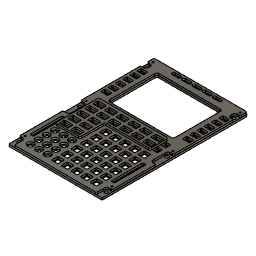
MCDU (3D layered extrusion based on SVG) (Autodesk Fusion 360 design; units mm, degrees)
Autodesk Fusion 360 part; units mm, degrees
(part 1 of 3)
sketch "Bottom" plane through (0, 0, 0) normal (0, 0, 1) x (1, 0, 0)
  ellipse E0 centre (25.7081, -64.7405) end of major axis (27.0103, -64.7405) minor radius 1.2936 (25.7081, -66.0341) -> (24.4058, -64.7405) cw
  line L0 (25.7081, -66.0341) -> (36.7769, -66.0341)
  ellipse E1 centre (36.7769, -64.7405) end of major axis (38.0792, -64.7405) minor radius 1.2936 (38.0792, -64.7405) -> (36.7769, -66.0341) cw
  line L1 (38.0792, -64.7405) -> (38.0792, -58.6604)
  ellipse E2 centre (36.7769, -58.6604) end of major axis (38.0792, -58.6604) minor radius 1.2936 (36.7769, -57.3667) -> (38.0792, -58.6604) cw
  line L2 (36.7769, -57.3667) -> (25.7081, -57.3667)
  ellipse E3 centre (25.7081, -58.6604) end of major axis (27.0103, -58.6604) minor radius 1.2936 (24.4058, -58.6604) -> (25.7081, -57.3667) cw
  line L3 (24.4058, -58.6604) -> (24.4058, -64.7405)
  ellipse E4 centre (25.7081, -75.9348) end of major axis (27.0103, -75.9348) minor radius 1.2936 (25.7081, -77.2285) -> (24.4058, -75.9348) cw
  line L4 (25.7081, -77.2285) -> (36.7769, -77.2285)
  ellipse E5 centre (36.7769, -75.9348) end of major axis (38.0792, -75.9348) minor radius 1.2936 (38.0792, -75.9348) -> (36.7769, -77.2285) cw
  line L5 (38.0792, -75.9348) -> (38.0792, -69.8548)
  ellipse E6 centre (36.7769, -69.8548) end of major axis (38.0792, -69.8548) minor radius 1.2936 (36.7769, -68.5611) -> (38.0792, -69.8548) cw
  line L6 (36.7769, -68.5611) -> (25.7081, -68.5611)
  ellipse E7 centre (25.7081, -69.8548) end of major axis (27.0103, -69.8548) minor radius 1.2936 (24.4058, -69.8548) -> (25.7081, -68.5611) cw
  line L7 (24.4058, -69.8548) -> (24.4058, -75.9348)
  ellipse E8 centre (25.7081, -87.174) end of major axis (27.0103, -87.174) minor radius 1.2936 (25.7081, -88.4676) -> (24.4058, -87.174) cw
  line L8 (25.7081, -88.4676) -> (36.7769, -88.4676)
  ellipse E9 centre (36.7769, -87.174) end of major axis (38.0792, -87.174) minor radius 1.2936 (38.0792, -87.174) -> (36.7769, -88.4676) cw
  line L9 (38.0792, -87.174) -> (38.0792, -81.0939)
  ellipse E10 centre (36.7769, -81.0939) end of major axis (38.0792, -81.0939) minor radius 1.2936 (36.7769, -79.8003) -> (38.0792, -81.0939) cw
  line L10 (36.7769, -79.8003) -> (25.7081, -79.8003)
  ellipse E11 centre (25.7081, -81.0939) end of major axis (27.0103, -81.0939) minor radius 1.2936 (24.4058, -81.0939) -> (25.7081, -79.8003) cw
  line L11 (24.4058, -81.0939) -> (24.4058, -87.174)
  ellipse E12 centre (25.7081, -98.4373) end of major axis (27.0103, -98.4373) minor radius 1.2936 (25.7081, -99.7309) -> (24.4058, -98.4373) cw
  line L12 (25.7081, -99.7309) -> (36.7769, -99.7309)
  ellipse E13 centre (36.7769, -98.4373) end of major axis (38.0792, -98.4373) minor radius 1.2936 (38.0792, -98.4373) -> (36.7769, -99.7309) cw
  line L13 (38.0792, -98.4373) -> (38.0792, -92.3572)
  ellipse E14 centre (36.7769, -92.3572) end of major axis (38.0792, -92.3572) minor radius 1.2936 (36.7769, -91.0636) -> (38.0792, -92.3572) cw
  line L14 (36.7769, -91.0636) -> (25.7081, -91.0636)
  ellipse E15 centre (25.7081, -92.3572) end of major axis (27.0103, -92.3572) minor radius 1.2936 (24.4058, -92.3572) -> (25.7081, -91.0636) cw
  line L15 (24.4058, -92.3572) -> (24.4058, -98.4373)
  ellipse E16 centre (25.7081, -109.6497) end of major axis (27.0103, -109.6497) minor radius 1.2936 (25.7081, -110.9433) -> (24.4058, -109.6497) cw
  line L16 (25.7081, -110.9433) -> (36.7769, -110.9433)
  ellipse E17 centre (36.7769, -109.6497) end of major axis (38.0792, -109.6497) minor radius 1.2936 (38.0792, -109.6497) -> (36.7769, -110.9433) cw
  line L17 (38.0792, -109.6497) -> (38.0792, -103.5696)
  ellipse E18 centre (36.7769, -103.5696) end of major axis (38.0792, -103.5696) minor radius 1.2936 (36.7769, -102.276) -> (38.0792, -103.5696) cw
  line L18 (36.7769, -102.276) -> (25.7081, -102.276)
  ellipse E19 centre (25.7081, -103.5696) end of major axis (27.0103, -103.5696) minor radius 1.2936 (24.4058, -103.5696) -> (25.7081, -102.276) cw
  line L19 (24.4058, -103.5696) -> (24.4058, -109.6497)
  ellipse E20 centre (25.7081, -120.8865) end of major axis (27.0103, -120.8865) minor radius 1.2936 (25.7081, -122.1801) -> (24.4058, -120.8865) cw
  line L20 (25.7081, -122.1801) -> (36.7769, -122.1801)
  ellipse E21 centre (36.7769, -120.8865) end of major axis (38.0792, -120.8865) minor radius 1.2936 (38.0792, -120.8865) -> (36.7769, -122.1801) cw
  line L21 (38.0792, -120.8865) -> (38.0792, -114.8064)
  ellipse E22 centre (36.7769, -114.8064) end of major axis (38.0792, -114.8064) minor radius 1.2936 (36.7769, -113.5127) -> (38.0792, -114.8064) cw
  line L22 (36.7769, -113.5127) -> (25.7081, -113.5127)
  ellipse E23 centre (25.7081, -114.8064) end of major axis (27.0103, -114.8064) minor radius 1.2936 (24.4058, -114.8064) -> (25.7081, -113.5127) cw
  line L23 (24.4058, -114.8064) -> (24.4058, -120.8865)
  ellipse E24 centre (153.6745, -120.9659) end of major axis (154.9767, -120.9659) minor radius 1.2936 (153.6745, -122.2596) -> (152.3723, -120.9659) cw
  line L24 (153.6745, -122.2596) -> (164.7434, -122.2596)
  ellipse E25 centre (164.7434, -120.9659) end of major axis (166.0456, -120.9659) minor radius 1.2936 (166.0456, -120.9659) -> (164.7434, -122.2596) cw
  line L25 (166.0456, -120.9659) -> (166.0456, -114.8858)
  ellipse E26 centre (164.7434, -114.8858) end of major axis (166.0456, -114.8858) minor radius 1.2936 (164.7434, -113.5922) -> (166.0456, -114.8858) cw
  line L26 (164.7434, -113.5922) -> (153.6745, -113.5922)
  ellipse E27 centre (153.6745, -114.8858) end of major axis (154.9767, -114.8858) minor radius 1.2936 (152.3723, -114.8858) -> (153.6745, -113.5922) cw
  line L27 (152.3723, -114.8858) -> (152.3723, -120.9659)
  ellipse E28 centre (153.6745, -98.4902) end of major axis (154.9767, -98.4902) minor radius 1.2936 (153.6745, -99.7839) -> (152.3723, -98.4902) cw
  line L28 (153.6745, -99.7839) -> (164.7434, -99.7839)
  ellipse E29 centre (164.7434, -98.4902) end of major axis (166.0456, -98.4902) minor radius 1.2936 (166.0456, -98.4902) -> (164.7434, -99.7839) cw
  line L29 (166.0456, -98.4902) -> (166.0456, -92.4102)
  ellipse E30 centre (164.7434, -92.4102) end of major axis (166.0456, -92.4102) minor radius 1.2936 (164.7434, -91.1165) -> (166.0456, -92.4102) cw
  line L30 (164.7434, -91.1165) -> (153.6745, -91.1165)
  ellipse E31 centre (153.6745, -92.4102) end of major axis (154.9767, -92.4102) minor radius 1.2936 (152.3723, -92.4102) -> (153.6745, -91.1165) cw
  line L31 (152.3723, -92.4102) -> (152.3723, -98.4902)
  ellipse E32 centre (153.6745, -87.28) end of major axis (154.9767, -87.28) minor radius 1.2936 (153.6745, -88.5736) -> (152.3723, -87.28) cw
  line L32 (153.6745, -88.5736) -> (164.7434, -88.5736)
  ellipse E33 centre (164.7434, -87.28) end of major axis (166.0456, -87.28) minor radius 1.2936 (166.0456, -87.28) -> (164.7434, -88.5736) cw
  line L33 (166.0456, -87.28) -> (166.0456, -81.1999)
  ellipse E34 centre (164.7434, -81.1999) end of major axis (166.0456, -81.1999) minor radius 1.2936 (164.7434, -79.9062) -> (166.0456, -81.1999) cw
  line L34 (164.7434, -79.9062) -> (153.6745, -79.9062)
  ellipse E35 centre (153.6745, -81.1999) end of major axis (154.9767, -81.1999) minor radius 1.2936 (152.3723, -81.1999) -> (153.6745, -79.9062) cw
  line L35 (152.3723, -81.1999) -> (152.3723, -87.28)
  ellipse E36 centre (153.6745, -76.0143) end of major axis (154.9767, -76.0143) minor radius 1.2936 (153.6745, -77.308) -> (152.3723, -76.0143) cw
  line L36 (153.6745, -77.308) -> (164.7434, -77.308)
  ellipse E37 centre (164.7434, -76.0143) end of major axis (166.0456, -76.0143) minor radius 1.2936 (166.0456, -76.0143) -> (164.7434, -77.308) cw
  line L37 (166.0456, -76.0143) -> (166.0456, -69.9342)
  ellipse E38 centre (164.7434, -69.9342) end of major axis (166.0456, -69.9342) minor radius 1.2936 (164.7434, -68.6406) -> (166.0456, -69.9342) cw
  line L38 (164.7434, -68.6406) -> (153.6745, -68.6406)
  ellipse E39 centre (153.6745, -69.9342) end of major axis (154.9767, -69.9342) minor radius 1.2936 (152.3723, -69.9342) -> (153.6745, -68.6406) cw
  line L39 (152.3723, -69.9342) -> (152.3723, -76.0143)
  ellipse E40 centre (153.6748, -64.7405) end of major axis (154.977, -64.7405) minor radius 1.2936 (153.6748, -66.0341) -> (152.3726, -64.7405) cw
  line L40 (153.6748, -66.0341) -> (164.7437, -66.0341)
  ellipse E41 centre (164.7437, -64.7405) end of major axis (166.0459, -64.7405) minor radius 1.2936 (166.0459, -64.7405) -> (164.7437, -66.0341) cw
  line L41 (166.0459, -64.7405) -> (166.0459, -58.6604)
  ellipse E42 centre (164.7437, -58.6604) end of major axis (166.0459, -58.6604) minor radius 1.2936 (164.7437, -57.3667) -> (166.0459, -58.6604) cw
  line L42 (164.7437, -57.3667) -> (153.6748, -57.3667)
  ellipse E43 centre (153.6748, -58.6604) end of major axis (154.977, -58.6604) minor radius 1.2936 (152.3726, -58.6604) -> (153.6748, -57.3667) cw
  line L43 (152.3726, -58.6604) -> (152.3726, -64.7405)
  ellipse E44 centre (39.5473, -146.6503) end of major axis (40.6602, -146.6503) minor radius 1.1983 (39.5473, -147.8487) -> (38.4344, -146.6503) cw
  line L44 (39.5473, -147.8487) -> (52.0339, -147.8487)
  ellipse E45 centre (52.0339, -146.6503) end of major axis (53.1468, -146.6503) minor radius 1.1983 (53.1468, -146.6503) -> (52.0339, -147.8487) cw
  line L45 (53.1468, -146.6503) -> (53.1468, -139.3406)
  ellipse E46 centre (52.0339, -139.3406) end of major axis (53.1468, -139.3406) minor radius 1.1983 (52.0339, -138.1423) -> (53.1468, -139.3406) cw
  line L46 (52.0339, -138.1423) -> (39.5473, -138.1423)
  ellipse E47 centre (39.5473, -139.3406) end of major axis (40.6602, -139.3406) minor radius 1.1983 (38.4344, -139.3406) -> (39.5473, -138.1423) cw
  line L47 (38.4344, -139.3406) -> (38.4344, -146.6503)
  ellipse E48 centre (39.5473, -159.4672) end of major axis (40.6602, -159.4672) minor radius 1.1983 (39.5473, -160.6656) -> (38.4344, -159.4672) cw
  line L48 (39.5473, -160.6656) -> (52.0339, -160.6656)
  ellipse E49 centre (52.0339, -159.4672) end of major axis (53.1468, -159.4672) minor radius 1.1983 (53.1468, -159.4672) -> (52.0339, -160.6656) cw
  line L49 (53.1468, -159.4672) -> (53.1468, -152.1575)
  ellipse E50 centre (52.0339, -152.1575) end of major axis (53.1468, -152.1575) minor radius 1.1983 (52.0339, -150.9592) -> (53.1468, -152.1575) cw
  line L50 (52.0339, -150.9592) -> (39.5473, -150.9592)
  ellipse E51 centre (39.5473, -152.1575) end of major axis (40.6602, -152.1575) minor radius 1.1983 (38.4344, -152.1575) -> (39.5473, -150.9592) cw
  line L51 (38.4344, -152.1575) -> (38.4344, -159.4672)
  ellipse E52 centre (39.5473, -172.8669) end of major axis (40.6602, -172.8669) minor radius 1.1983 (39.5473, -174.0652) -> (38.4344, -172.8669) cw
  line L52 (39.5473, -174.0652) -> (52.0339, -174.0652)
  ellipse E53 centre (52.0339, -172.8669) end of major axis (53.1468, -172.8669) minor radius 1.1983 (53.1468, -172.8669) -> (52.0339, -174.0652) cw
  line L53 (53.1468, -172.8669) -> (53.1468, -165.5572)
  ellipse E54 centre (52.0339, -165.5572) end of major axis (53.1468, -165.5572) minor radius 1.1983 (52.0339, -164.3588) -> (53.1468, -165.5572) cw
  line L54 (52.0339, -164.3588) -> (39.5473, -164.3588)
  ellipse E55 centre (39.5473, -165.5572) end of major axis (40.6602, -165.5572) minor radius 1.1983 (38.4344, -165.5572) -> (39.5473, -164.3588) cw
  line L55 (38.4344, -165.5572) -> (38.4344, -172.8669)
  ellipse E56 centre (39.5473, -185.9547) end of major axis (40.6602, -185.9547) minor radius 1.1983 (39.5473, -187.1531) -> (38.4344, -185.9547) cw
  line L56 (39.5473, -187.1531) -> (52.0339, -187.1531)
  ellipse E57 centre (52.0339, -185.9547) end of major axis (53.1468, -185.9547) minor radius 1.1983 (53.1468, -185.9547) -> (52.0339, -187.1531) cw
  line L57 (53.1468, -185.9547) -> (53.1468, -178.645)
  ellipse E58 centre (52.0339, -178.645) end of major axis (53.1468, -178.645) minor radius 1.1983 (52.0339, -177.4467) -> (53.1468, -178.645) cw
  line L58 (52.0339, -177.4467) -> (39.5473, -177.4466)
  ellipse E59 centre (39.5473, -178.645) end of major axis (40.6602, -178.645) minor radius 1.1983 (38.4344, -178.645) -> (39.5473, -177.4466) cw
  line L59 (38.4344, -178.645) -> (38.4344, -185.9547)
  ellipse E60 centre (39.5473, -198.9895) end of major axis (40.6602, -198.9895) minor radius 1.1983 (39.5473, -200.1878) -> (38.4344, -198.9895) cw
  line L60 (39.5473, -200.1878) -> (52.0339, -200.1878)
  ellipse E61 centre (52.0339, -198.9895) end of major axis (53.1468, -198.9895) minor radius 1.1983 (53.1468, -198.9895) -> (52.0339, -200.1878) cw
  line L61 (53.1468, -198.9895) -> (53.1468, -191.6797)
  ellipse E62 centre (52.0339, -191.6797) end of major axis (53.1468, -191.6797) minor radius 1.1983 (52.0339, -190.4814) -> (53.1468, -191.6797) cw
  line L62 (52.0339, -190.4814) -> (39.5473, -190.4814)
  ellipse E63 centre (39.5473, -191.6797) end of major axis (40.6602, -191.6797) minor radius 1.1983 (38.4344, -191.6797) -> (39.5473, -190.4814) cw
  line L63 (38.4344, -191.6797) -> (38.4344, -198.9895)
  ellipse E64 centre (57.4439, -198.9895) end of major axis (58.5568, -198.9895) minor radius 1.1983 (57.4439, -200.1878) -> (56.331, -198.9895) cw
  line L64 (57.4439, -200.1878) -> (69.9305, -200.1878)
  ellipse E65 centre (69.9305, -198.9895) end of major axis (71.0434, -198.9895) minor radius 1.1983 (71.0434, -198.9895) -> (69.9305, -200.1878) cw
  line L65 (71.0434, -198.9895) -> (71.0434, -191.6797)
  ellipse E66 centre (69.9305, -191.6797) end of major axis (71.0434, -191.6797) minor radius 1.1983 (69.9305, -190.4814) -> (71.0434, -191.6797) cw
  line L66 (69.9305, -190.4814) -> (57.4439, -190.4814)
  ellipse E67 centre (57.4439, -191.6797) end of major axis (58.5568, -191.6797) minor radius 1.1983 (56.331, -191.6797) -> (57.4439, -190.4814) cw
  line L67 (56.331, -191.6797) -> (56.331, -198.9895)
  ellipse E68 centre (57.4439, -185.9547) end of major axis (58.5568, -185.9547) minor radius 1.1983 (57.4439, -187.1531) -> (56.331, -185.9547) cw
  line L68 (57.4439, -187.1531) -> (69.9305, -187.1531)
  ellipse E69 centre (69.9305, -185.9547) end of major axis (71.0434, -185.9547) minor radius 1.1983 (71.0434, -185.9547) -> (69.9305, -187.1531) cw
  line L69 (71.0434, -185.9547) -> (71.0434, -178.645)
  ellipse E70 centre (69.9305, -178.645) end of major axis (71.0434, -178.645) minor radius 1.1983 (69.9305, -177.4467) -> (71.0434, -178.645) cw
  line L70 (69.9305, -177.4467) -> (57.4439, -177.4466)
  ellipse E71 centre (57.4439, -178.645) end of major axis (58.5568, -178.645) minor radius 1.1983 (56.331, -178.645) -> (57.4439, -177.4466) cw
  line L71 (56.331, -178.645) -> (56.331, -185.9547)
  ellipse E72 centre (57.4439, -172.8669) end of major axis (58.5568, -172.8669) minor radius 1.1983 (57.4439, -174.0652) -> (56.331, -172.8669) cw
  line L72 (57.4439, -174.0652) -> (69.9305, -174.0652)
  ellipse E73 centre (69.9305, -172.8669) end of major axis (71.0434, -172.8669) minor radius 1.1983 (71.0434, -172.8669) -> (69.9305, -174.0652) cw
  line L73 (71.0434, -172.8669) -> (71.0434, -165.5572)
  ellipse E74 centre (69.9305, -165.5572) end of major axis (71.0434, -165.5572) minor radius 1.1983 (69.9305, -164.3588) -> (71.0434, -165.5572) cw
  line L74 (69.9305, -164.3588) -> (57.4439, -164.3588)
  ellipse E75 centre (57.4439, -165.5572) end of major axis (58.5568, -165.5572) minor radius 1.1983 (56.331, -165.5572) -> (57.4439, -164.3588) cw
  line L75 (56.331, -165.5572) -> (56.331, -172.8669)
  ellipse E76 centre (57.4439, -159.4672) end of major axis (58.5568, -159.4672) minor radius 1.1983 (57.4439, -160.6656) -> (56.331, -159.4672) cw
  line L76 (57.4439, -160.6656) -> (69.9305, -160.6656)
  ellipse E77 centre (69.9305, -159.4672) end of major axis (71.0434, -159.4672) minor radius 1.1983 (71.0434, -159.4672) -> (69.9305, -160.6656) cw
  line L77 (71.0434, -159.4672) -> (71.0434, -152.1575)
  ellipse E78 centre (69.9305, -152.1575) end of major axis (71.0434, -152.1575) minor radius 1.1983 (69.9305, -150.9592) -> (71.0434, -152.1575) cw
  line L78 (69.9305, -150.9592) -> (57.4439, -150.9592)
  ellipse E79 centre (57.4439, -152.1575) end of major axis (58.5568, -152.1575) minor radius 1.1983 (56.331, -152.1575) -> (57.4439, -150.9592) cw
  line L79 (56.331, -152.1575) -> (56.331, -159.4672)
  ellipse E80 centre (57.4439, -146.6503) end of major axis (58.5568, -146.6503) minor radius 1.1983 (57.4439, -147.8487) -> (56.331, -146.6503) cw
  line L80 (57.4439, -147.8487) -> (69.9305, -147.8487)
  ellipse E81 centre (69.9305, -146.6503) end of major axis (71.0434, -146.6503) minor radius 1.1983 (71.0434, -146.6503) -> (69.9305, -147.8487) cw
  line L81 (71.0434, -146.6503) -> (71.0434, -139.3406)
  ellipse E82 centre (69.9305, -139.3406) end of major axis (71.0434, -139.3406) minor radius 1.1983 (69.9305, -138.1423) -> (71.0434, -139.3406) cw
  line L82 (69.9305, -138.1423) -> (57.4439, -138.1423)
  ellipse E83 centre (57.4439, -139.3406) end of major axis (58.5568, -139.3406) minor radius 1.1983 (56.331, -139.3406) -> (57.4439, -138.1423) cw
  line L83 (56.331, -139.3406) -> (56.331, -146.6503)
  ellipse E84 centre (75.6043, -146.6503) end of major axis (76.7172, -146.6503) minor radius 1.1983 (75.6044, -147.8487) -> (74.4915, -146.6503) cw
  line L84 (75.6044, -147.8487) -> (88.091, -147.8487)
  ellipse E85 centre (88.0909, -146.6503) end of major axis (89.2038, -146.6503) minor radius 1.1983 (89.2038, -146.6503) -> (88.091, -147.8487) cw
  line L85 (89.2038, -146.6503) -> (89.2038, -139.3406)
  ellipse E86 centre (88.0909, -139.3406) end of major axis (89.2038, -139.3406) minor radius 1.1983 (88.091, -138.1423) -> (89.2038, -139.3406) cw
  line L86 (88.091, -138.1423) -> (75.6044, -138.1423)
  ellipse E87 centre (75.6043, -139.3406) end of major axis (76.7172, -139.3406) minor radius 1.1983 (74.4915, -139.3406) -> (75.6044, -138.1423) cw
  line L87 (74.4915, -139.3406) -> (74.4915, -146.6503)
  ellipse E88 centre (75.6043, -159.4672) end of major axis (76.7172, -159.4672) minor radius 1.1983 (75.6044, -160.6656) -> (74.4915, -159.4672) cw
  line L88 (75.6044, -160.6656) -> (88.091, -160.6656)
  ellipse E89 centre (88.0909, -159.4672) end of major axis (89.2038, -159.4672) minor radius 1.1983 (89.2038, -159.4672) -> (88.091, -160.6656) cw
  line L89 (89.2038, -159.4672) -> (89.2038, -152.1575)
  ellipse E90 centre (88.0909, -152.1575) end of major axis (89.2038, -152.1575) minor radius 1.1983 (88.091, -150.9592) -> (89.2038, -152.1575) cw
  line L90 (88.091, -150.9592) -> (75.6044, -150.9592)
  ellipse E91 centre (75.6043, -152.1575) end of major axis (76.7172, -152.1575) minor radius 1.1983 (74.4915, -152.1575) -> (75.6044, -150.9592) cw
  line L91 (74.4915, -152.1575) -> (74.4915, -159.4672)
  ellipse E92 centre (93.7913, -146.6503) end of major axis (94.9042, -146.6503) minor radius 1.1983 (93.7913, -147.8487) -> (92.6784, -146.6503) cw
  line L92 (93.7913, -147.8487) -> (106.2779, -147.8487)
  ellipse E93 centre (106.2779, -146.6503) end of major axis (107.3908, -146.6503) minor radius 1.1983 (107.3908, -146.6503) -> (106.2779, -147.8487) cw
  line L93 (107.3908, -146.6503) -> (107.3908, -139.3406)
  ellipse E94 centre (106.2779, -139.3406) end of major axis (107.3908, -139.3406) minor radius 1.1983 (106.2779, -138.1423) -> (107.3908, -139.3406) cw
  line L94 (106.2779, -138.1423) -> (93.7913, -138.1423)
  ellipse E95 centre (93.7913, -139.3406) end of major axis (94.9042, -139.3406) minor radius 1.1983 (92.6784, -139.3406) -> (93.7913, -138.1423) cw
  line L95 (92.6784, -139.3406) -> (92.6784, -146.6503)
  ellipse E96 centre (93.7913, -159.4672) end of major axis (94.9042, -159.4672) minor radius 1.1983 (93.7913, -160.6656) -> (92.6784, -159.4672) cw
  line L96 (93.7913, -160.6656) -> (106.2779, -160.6656)
  ellipse E97 centre (106.2779, -159.4672) end of major axis (107.3908, -159.4672) minor radius 1.1983 (107.3908, -159.4672) -> (106.2779, -160.6656) cw
  line L97 (107.3908, -159.4672) -> (107.3908, -152.1575)
  ellipse E98 centre (106.2779, -152.1575) end of major axis (107.3908, -152.1575) minor radius 1.1983 (106.2779, -150.9592) -> (107.3908, -152.1575) cw
  line L98 (106.2779, -150.9592) -> (93.7913, -150.9592)
  ellipse E99 centre (93.7913, -152.1575) end of major axis (94.9042, -152.1575) minor radius 1.1983 (92.6784, -152.1575) -> (93.7913, -150.9592) cw
  line L99 (92.6784, -152.1575) -> (92.6784, -159.4672)
  ellipse E100 centre (111.7928, -146.6503) end of major axis (112.9057, -146.6503) minor radius 1.1983 (111.7928, -147.8487) -> (110.6799, -146.6503) cw
  line L100 (111.7928, -147.8487) -> (124.2794, -147.8487)
  ellipse E101 centre (124.2794, -146.6503) end of major axis (125.3923, -146.6503) minor radius 1.1983 (125.3923, -146.6503) -> (124.2794, -147.8487) cw
  line L101 (125.3923, -146.6503) -> (125.3923, -139.3406)
  ellipse E102 centre (124.2794, -139.3406) end of major axis (125.3923, -139.3406) minor radius 1.1983 (124.2794, -138.1423) -> (125.3923, -139.3406) cw
  line L102 (124.2794, -138.1423) -> (111.7928, -138.1423)
  ellipse E103 centre (111.7928, -139.3406) end of major axis (112.9057, -139.3406) minor radius 1.1983 (110.6799, -139.3406) -> (111.7928, -138.1423) cw
  line L103 (110.6799, -139.3406) -> (110.6799, -146.6503)
  ellipse E104 centre (111.7928, -159.4672) end of major axis (112.9057, -159.4672) minor radius 1.1983 (111.7928, -160.6656) -> (110.6799, -159.4672) cw
  line L104 (111.7928, -160.6656) -> (124.2794, -160.6656)
  ellipse E105 centre (124.2794, -159.4672) end of major axis (125.3923, -159.4672) minor radius 1.1983 (125.3923, -159.4672) -> (124.2794, -160.6656) cw
  line L105 (125.3923, -159.4672) -> (125.3923, -152.1575)
  ellipse E106 centre (124.2794, -152.1575) end of major axis (125.3923, -152.1575) minor radius 1.1983 (124.2794, -150.9592) -> (125.3923, -152.1575) cw
  line L106 (124.2794, -150.9592) -> (111.7928, -150.9592)
  ellipse E107 centre (111.7928, -152.1575) end of major axis (112.9057, -152.1575) minor radius 1.1983 (110.6799, -152.1575) -> (111.7928, -150.9592) cw
  line L107 (110.6799, -152.1575) -> (110.6799, -159.4672)
  ellipse E108 centre (129.7572, -146.6503) end of major axis (130.8701, -146.6503) minor radius 1.1983 (129.7572, -147.8487) -> (128.6444, -146.6503) cw
  line L108 (129.7572, -147.8487) -> (142.2439, -147.8487)
  ellipse E109 centre (142.2439, -146.6503) end of major axis (143.3567, -146.6503) minor radius 1.1983 (143.3567, -146.6503) -> (142.2439, -147.8487) cw
  line L109 (143.3567, -146.6503) -> (143.3567, -139.3406)
  ellipse E110 centre (142.2439, -139.3406) end of major axis (143.3567, -139.3406) minor radius 1.1983 (142.2439, -138.1423) -> (143.3567, -139.3406) cw
  line L110 (142.2439, -138.1423) -> (129.7573, -138.1423)
  ellipse E111 centre (129.7573, -139.3406) end of major axis (130.8701, -139.3406) minor radius 1.1983 (128.6444, -139.3406) -> (129.7573, -138.1423) cw
  line L111 (128.6444, -139.3406) -> (128.6444, -146.6503)
  ellipse E112 centre (129.7572, -159.4672) end of major axis (130.8701, -159.4672) minor radius 1.1983 (129.7572, -160.6656) -> (128.6444, -159.4672) cw
  line L112 (129.7572, -160.6656) -> (142.2439, -160.6656)
  ellipse E113 centre (142.2439, -159.4672) end of major axis (143.3567, -159.4672) minor radius 1.1983 (143.3567, -159.4672) -> (142.2439, -160.6656) cw
  line L113 (143.3567, -159.4672) -> (143.3567, -152.1575)
  ellipse E114 centre (142.2439, -152.1575) end of major axis (143.3567, -152.1575) minor radius 1.1983 (142.2439, -150.9592) -> (143.3567, -152.1575) cw
  line L114 (142.2439, -150.9592) -> (129.7573, -150.9592)
  ellipse E115 centre (129.7573, -152.1575) end of major axis (130.8701, -152.1575) minor radius 1.1983 (128.6444, -152.1575) -> (129.7573, -150.9592) cw
  line L115 (128.6444, -152.1575) -> (128.6444, -159.4672)
  arc A0 (125.3436, -178.7576) -> (124.0756, -177.4896) centre (125.3436, -177.4896) cw
  line L116 (125.3436, -178.7576) -> (135.4877, -178.7576)
  arc A1 (136.7557, -177.4896) -> (135.4877, -178.7576) centre (135.4877, -177.4896) cw
  line L117 (136.7557, -177.4896) -> (136.7557, -167.3456)
  arc A2 (135.4877, -166.0776) -> (136.7557, -167.3456) centre (135.4877, -167.3456) cw
  line L118 (135.4877, -166.0776) -> (125.3436, -166.0776)
  arc A3 (124.0756, -167.3456) -> (125.3436, -166.0776) centre (125.3436, -167.3456) cw
  line L119 (124.0756, -167.3456) -> (124.0756, -177.4896)
  arc A4 (140.3318, -178.7166) -> (139.0637, -177.4486) centre (140.3317, -177.4486) cw
  line L120 (140.3318, -178.7166) -> (150.4758, -178.7166)
  arc A5 (151.7438, -177.4486) -> (150.4758, -178.7166) centre (150.4758, -177.4486) cw
  line L121 (151.7438, -177.4486) -> (151.7438, -167.3045)
  arc A6 (150.4758, -166.0365) -> (151.7438, -167.3045) centre (150.4758, -167.3045) cw
  line L122 (150.4758, -166.0365) -> (140.3318, -166.0365)
  arc A7 (139.0638, -167.3045) -> (140.3318, -166.0365) centre (140.3318, -167.3045) cw
  line L123 (139.0638, -167.3045) -> (139.0637, -177.4486)
  arc A8 (80.0241, -178.7576) -> (78.7561, -177.4896) centre (80.0241, -177.4896) cw
  line L124 (80.0241, -178.7576) -> (90.1681, -178.7576)
  arc A9 (91.4361, -177.4896) -> (90.1681, -178.7576) centre (90.1681, -177.4896) cw
  line L125 (91.4361, -177.4896) -> (91.4361, -167.3456)
  arc A10 (90.1681, -166.0776) -> (91.4361, -167.3456) centre (90.1681, -167.3456) cw
  line L126 (90.1681, -166.0776) -> (80.0241, -166.0776)
  arc A11 (78.7561, -167.3456) -> (80.0241, -166.0776) centre (80.0241, -167.3456) cw
  line L127 (78.7561, -167.3456) -> (78.7561, -177.4896)
  arc A12 (95.0489, -178.7576) -> (93.7809, -177.4896) centre (95.0489, -177.4896) cw
  line L128 (95.0489, -178.7576) -> (105.193, -178.7576)
  arc A13 (106.461, -177.4896) -> (105.193, -178.7576) centre (105.193, -177.4896) cw
  line L129 (106.461, -177.4896) -> (106.461, -167.3456)
  arc A14 (105.193, -166.0776) -> (106.461, -167.3456) centre (105.193, -167.3456) cw
  line L130 (105.193, -166.0776) -> (95.0489, -166.0776)
  arc A15 (93.7809, -167.3456) -> (95.0489, -166.0776) centre (95.0489, -167.3456) cw
  line L131 (93.7809, -167.3456) -> (93.7809, -177.4896)
  arc A16 (110.2136, -178.7576) -> (108.9456, -177.4896) centre (110.2136, -177.4896) cw
  line L132 (110.2136, -178.7576) -> (120.3577, -178.7576)
  arc A17 (121.6257, -177.4896) -> (120.3577, -178.7576) centre (120.3577, -177.4896) cw
  line L133 (121.6257, -177.4896) -> (121.6257, -167.3456)
  arc A18 (120.3577, -166.0776) -> (121.6257, -167.3456) centre (120.3577, -167.3456) cw
  line L134 (120.3577, -166.0776) -> (110.2136, -166.0776)
  arc A19 (108.9456, -167.3456) -> (110.2136, -166.0776) centre (110.2136, -167.3456) cw
  line L135 (108.9456, -167.3456) -> (108.9456, -177.4896)
  arc A20 (140.3318, -193.6928) -> (139.0637, -192.4248) centre (140.3317, -192.4248) cw
  line L136 (140.3318, -193.6928) -> (150.4758, -193.6928)
  arc A21 (151.7438, -192.4248) -> (150.4758, -193.6928) centre (150.4758, -192.4248) cw
  line L137 (151.7438, -192.4248) -> (151.7438, -182.2807)
  arc A22 (150.4758, -181.0127) -> (151.7438, -182.2807) centre (150.4758, -182.2807) cw
  line L138 (150.4758, -181.0127) -> (140.3318, -181.0127)
  arc A23 (139.0638, -182.2807) -> (140.3318, -181.0127) centre (140.3318, -182.2807) cw
  line L139 (139.0638, -182.2807) -> (139.0637, -192.4248)
  arc A24 (125.3436, -193.7338) -> (124.0756, -192.4658) centre (125.3436, -192.4658) cw
  line L140 (125.3436, -193.7338) -> (135.4877, -193.7338)
  arc A25 (136.7557, -192.4658) -> (135.4877, -193.7338) centre (135.4877, -192.4658) cw
  line L141 (136.7557, -192.4658) -> (136.7557, -182.3218)
  arc A26 (135.4877, -181.0538) -> (136.7557, -182.3218) centre (135.4877, -182.3218) cw
  line L142 (135.4877, -181.0538) -> (125.3436, -181.0538)
  arc A27 (124.0756, -182.3218) -> (125.3436, -181.0538) centre (125.3436, -182.3218) cw
  line L143 (124.0756, -182.3218) -> (124.0756, -192.4658)
  arc A28 (110.2136, -193.7338) -> (108.9456, -192.4658) centre (110.2136, -192.4658) cw
  line L144 (110.2136, -193.7338) -> (120.3577, -193.7338)
  arc A29 (121.6257, -192.4658) -> (120.3577, -193.7338) centre (120.3577, -192.4658) cw
  line L145 (121.6257, -192.4658) -> (121.6257, -182.3218)
  arc A30 (120.3577, -181.0538) -> (121.6257, -182.3218) centre (120.3577, -182.3218) cw
  line L146 (120.3577, -181.0538) -> (110.2136, -181.0538)
  arc A31 (108.9456, -182.3218) -> (110.2136, -181.0538) centre (110.2136, -182.3218) cw
  line L147 (108.9456, -182.3218) -> (108.9456, -192.4658)
  arc A32 (95.0489, -193.7338) -> (93.7809, -192.4658) centre (95.0489, -192.4658) cw
  line L148 (95.0489, -193.7338) -> (105.193, -193.7338)
  arc A33 (106.461, -192.4658) -> (105.193, -193.7338) centre (105.193, -192.4658) cw
  line L149 (106.461, -192.4658) -> (106.461, -182.3218)
  arc A34 (105.193, -181.0538) -> (106.461, -182.3218) centre (105.193, -182.3218) cw
  line L150 (105.193, -181.0538) -> (95.0489, -181.0538)
  arc A35 (93.7809, -182.3218) -> (95.0489, -181.0538) centre (95.0489, -182.3218) cw
  line L151 (93.7809, -182.3218) -> (93.7809, -192.4658)
  arc A36 (80.0241, -193.7338) -> (78.7561, -192.4658) centre (80.0241, -192.4658) cw
  line L152 (80.0241, -193.7338) -> (90.1681, -193.7338)
  arc A37 (91.4361, -192.4658) -> (90.1681, -193.7338) centre (90.1681, -192.4658) cw
  line L153 (91.4361, -192.4658) -> (91.4361, -182.3218)
  arc A38 (90.1681, -181.0538) -> (91.4361, -182.3218) centre (90.1681, -182.3218) cw
  line L154 (90.1681, -181.0538) -> (80.0241, -181.0538)
  arc A39 (78.7561, -182.3218) -> (80.0241, -181.0538) centre (80.0241, -182.3218) cw
  line L155 (78.7561, -182.3218) -> (78.7561, -192.4658)
  arc A40 (140.3318, -208.7485) -> (139.0638, -207.4805) centre (140.3318, -207.4805) cw
  line L156 (140.3318, -208.7485) -> (150.4758, -208.7485)
  arc A41 (151.7438, -207.4805) -> (150.4758, -208.7485) centre (150.4758, -207.4805) cw
  line L157 (151.7438, -207.4805) -> (151.7438, -197.3365)
  arc A42 (150.4758, -196.0685) -> (151.7438, -197.3365) centre (150.4758, -197.3365) cw
  line L158 (150.4758, -196.0685) -> (140.3318, -196.0685)
  arc A43 (139.0638, -197.3365) -> (140.3318, -196.0685) centre (140.3318, -197.3365) cw
  line L159 (139.0638, -197.3365) -> (139.0638, -207.4805)
  arc A44 (125.3436, -208.7896) -> (124.0756, -207.5215) centre (125.3436, -207.5216) cw
  line L160 (125.3436, -208.7896) -> (135.4877, -208.7896)
  arc A45 (136.7557, -207.5215) -> (135.4877, -208.7896) centre (135.4877, -207.5216) cw
  line L161 (136.7557, -207.5215) -> (136.7557, -197.3775)
  arc A46 (135.4877, -196.1095) -> (136.7557, -197.3775) centre (135.4877, -197.3775) cw
  line L162 (135.4877, -196.1095) -> (125.3436, -196.1095)
  arc A47 (124.0756, -197.3775) -> (125.3436, -196.1095) centre (125.3436, -197.3775) cw
  line L163 (124.0756, -197.3775) -> (124.0756, -207.5215)
  arc A48 (110.2136, -208.7896) -> (108.9456, -207.5215) centre (110.2136, -207.5216) cw
  line L164 (110.2136, -208.7896) -> (120.3577, -208.7896)
  arc A49 (121.6257, -207.5215) -> (120.3577, -208.7896) centre (120.3577, -207.5216) cw
  line L165 (121.6257, -207.5215) -> (121.6257, -197.3775)
  arc A50 (120.3577, -196.1095) -> (121.6257, -197.3775) centre (120.3577, -197.3775) cw
  line L166 (120.3577, -196.1095) -> (110.2136, -196.1095)
  arc A51 (108.9456, -197.3775) -> (110.2136, -196.1095) centre (110.2136, -197.3775) cw
  line L167 (108.9456, -197.3775) -> (108.9456, -207.5215)
  arc A52 (95.0489, -208.7896) -> (93.7809, -207.5215) centre (95.0489, -207.5216) cw
  line L168 (95.0489, -208.7896) -> (105.193, -208.7896)
  arc A53 (106.461, -207.5215) -> (105.193, -208.7896) centre (105.193, -207.5216) cw
  line L169 (106.461, -207.5215) -> (106.461, -197.3775)
  arc A54 (105.193, -196.1095) -> (106.461, -197.3775) centre (105.193, -197.3775) cw
  line L170 (105.193, -196.1095) -> (95.0489, -196.1095)
  arc A55 (93.7809, -197.3775) -> (95.0489, -196.1095) centre (95.0489, -197.3775) cw
  line L171 (93.7809, -197.3775) -> (93.7809, -207.5215)
  arc A56 (80.0241, -208.7896) -> (78.7561, -207.5215) centre (80.0241, -207.5216) cw
  line L172 (80.0241, -208.7896) -> (90.1681, -208.7896)
  arc A57 (91.4361, -207.5215) -> (90.1681, -208.7896) centre (90.1681, -207.5216) cw
  line L173 (91.4361, -207.5215) -> (91.4361, -197.3775)
  arc A58 (90.1681, -196.1095) -> (91.4361, -197.3775) centre (90.1681, -197.3775) cw
  line L174 (90.1681, -196.1095) -> (80.0241, -196.1095)
  arc A59 (78.7561, -197.3775) -> (80.0241, -196.1095) centre (80.0241, -197.3775) cw
  line L175 (78.7561, -197.3775) -> (78.7561, -207.5215)
  arc A60 (140.3318, -223.7776) -> (139.0638, -222.5096) centre (140.3318, -222.5096) cw
  line L176 (140.3318, -223.7776) -> (150.4758, -223.7776)
  arc A61 (151.7438, -222.5096) -> (150.4758, -223.7776) centre (150.4758, -222.5096) cw
  line L177 (151.7438, -222.5096) -> (151.7438, -212.3655)
  arc A62 (150.4758, -211.0975) -> (151.7438, -212.3655) centre (150.4758, -212.3655) cw
  line L178 (150.4758, -211.0975) -> (140.3318, -211.0975)
  arc A63 (139.0638, -212.3655) -> (140.3318, -211.0975) centre (140.3318, -212.3655) cw
  line L179 (139.0638, -212.3655) -> (139.0638, -222.5096)
  arc A64 (125.3436, -223.8186) -> (124.0756, -222.5506) centre (125.3436, -222.5506) cw
  line L180 (125.3436, -223.8186) -> (135.4877, -223.8186)
  arc A65 (136.7557, -222.5506) -> (135.4877, -223.8186) centre (135.4877, -222.5506) cw
  line L181 (136.7557, -222.5506) -> (136.7557, -212.4066)
  arc A66 (135.4877, -211.1386) -> (136.7557, -212.4066) centre (135.4877, -212.4066) cw
  line L182 (135.4877, -211.1386) -> (125.3436, -211.1386)
  arc A67 (124.0756, -212.4066) -> (125.3436, -211.1386) centre (125.3436, -212.4066) cw
  line L183 (124.0756, -212.4066) -> (124.0756, -222.5506)
  arc A68 (110.2136, -223.8186) -> (108.9456, -222.5506) centre (110.2136, -222.5506) cw
  line L184 (110.2136, -223.8186) -> (120.3577, -223.8186)
  arc A69 (121.6257, -222.5506) -> (120.3577, -223.8186) centre (120.3577, -222.5506) cw
  line L185 (121.6257, -222.5506) -> (121.6257, -212.4066)
  arc A70 (120.3577, -211.1386) -> (121.6257, -212.4066) centre (120.3577, -212.4066) cw
  line L186 (120.3577, -211.1386) -> (110.2136, -211.1386)
  arc A71 (108.9456, -212.4066) -> (110.2136, -211.1386) centre (110.2136, -212.4066) cw
  line L187 (108.9456, -212.4066) -> (108.9456, -222.5506)
  arc A72 (95.0489, -223.8186) -> (93.7809, -222.5506) centre (95.0489, -222.5506) cw
  line L188 (95.0489, -223.8186) -> (105.193, -223.8186)
  arc A73 (106.461, -222.5506) -> (105.193, -223.8186) centre (105.193, -222.5506) cw
  line L189 (106.461, -222.5506) -> (106.461, -212.4066)
  arc A74 (105.193, -211.1386) -> (106.461, -212.4066) centre (105.193, -212.4066) cw
  line L190 (105.193, -211.1386) -> (95.0489, -211.1386)
  arc A75 (93.7809, -212.4066) -> (95.0489, -211.1386) centre (95.0489, -212.4066) cw
  line L191 (93.7809, -212.4066) -> (93.7809, -222.5506)
  arc A76 (80.0241, -223.8186) -> (78.7561, -222.5506) centre (80.0241, -222.5506) cw
  line L192 (80.0241, -223.8186) -> (90.1681, -223.8186)
  arc A77 (91.4361, -222.5506) -> (90.1681, -223.8186) centre (90.1681, -222.5506) cw
  line L193 (91.4361, -222.5506) -> (91.4361, -212.4066)
  arc A78 (90.1681, -211.1386) -> (91.4361, -212.4066) centre (90.1681, -212.4066) cw
  line L194 (90.1681, -211.1386) -> (80.0241, -211.1386)
  arc A79 (78.7561, -212.4066) -> (80.0241, -211.1386) centre (80.0241, -212.4066) cw
  line L195 (78.7561, -212.4066) -> (78.7561, -222.5506)
  arc A80 (140.3317, -238.8069) -> (139.0637, -237.5389) centre (140.3317, -237.5389) cw
  line L196 (140.3317, -238.8069) -> (150.4758, -238.8069)
  arc A81 (151.7438, -237.5389) -> (150.4758, -238.8069) centre (150.4758, -237.5389) cw
  line L197 (151.7438, -237.5389) -> (151.7438, -227.3949)
  arc A82 (150.4758, -226.1269) -> (151.7438, -227.3949) centre (150.4758, -227.3949) cw
  line L198 (150.4758, -226.1269) -> (140.3317, -226.1269)
  arc A83 (139.0637, -227.3949) -> (140.3317, -226.1269) centre (140.3317, -227.3949) cw
  line L199 (139.0637, -227.3949) -> (139.0637, -237.5389)
  arc A84 (125.3436, -238.848) -> (124.0756, -237.58) centre (125.3436, -237.58) cw
  line L200 (125.3436, -238.848) -> (135.4877, -238.848)
  arc A85 (136.7557, -237.58) -> (135.4877, -238.848) centre (135.4877, -237.58) cw
  line L201 (136.7557, -237.58) -> (136.7557, -227.4359)
  arc A86 (135.4877, -226.1679) -> (136.7557, -227.4359) centre (135.4877, -227.4359) cw
  line L202 (135.4877, -226.1679) -> (125.3436, -226.1679)
  arc A87 (124.0756, -227.436) -> (125.3436, -226.1679) centre (125.3436, -227.4359) cw
  line L203 (124.0756, -227.436) -> (124.0756, -237.58)
  arc A88 (110.2136, -238.848) -> (108.9456, -237.58) centre (110.2136, -237.58) cw
  line L204 (110.2136, -238.848) -> (120.3577, -238.848)
  arc A89 (121.6257, -237.58) -> (120.3577, -238.848) centre (120.3577, -237.58) cw
  line L205 (121.6257, -237.58) -> (121.6257, -227.4359)
  arc A90 (120.3577, -226.1679) -> (121.6257, -227.4359) centre (120.3577, -227.4359) cw
  line L206 (120.3577, -226.1679) -> (110.2136, -226.1679)
  arc A91 (108.9456, -227.436) -> (110.2136, -226.1679) centre (110.2136, -227.4359) cw
  line L207 (108.9456, -227.436) -> (108.9456, -237.58)
  arc A92 (95.0489, -238.848) -> (93.7809, -237.58) centre (95.0489, -237.58) cw
  line L208 (95.0489, -238.848) -> (105.193, -238.848)
  arc A93 (106.461, -237.58) -> (105.193, -238.848) centre (105.193, -237.58) cw
  line L209 (106.461, -237.58) -> (106.461, -227.4359)
  arc A94 (105.193, -226.1679) -> (106.461, -227.4359) centre (105.193, -227.4359) cw
  line L210 (105.193, -226.1679) -> (95.0489, -226.1679)
  arc A95 (93.7809, -227.436) -> (95.0489, -226.1679) centre (95.0489, -227.4359) cw
  line L211 (93.7809, -227.436) -> (93.7809, -237.58)
  arc A96 (80.0241, -238.848) -> (78.7561, -237.58) centre (80.0241, -237.58) cw
  line L212 (80.0241, -238.848) -> (90.1681, -238.848)
  arc A97 (91.4361, -237.58) -> (90.1681, -238.848) centre (90.1681, -237.58) cw
  line L213 (91.4361, -237.58) -> (91.4361, -227.4359)
  arc A98 (90.1681, -226.1679) -> (91.4361, -227.4359) centre (90.1681, -227.4359) cw
  line L214 (90.1681, -226.1679) -> (80.0241, -226.1679)
  arc A99 (78.7561, -227.436) -> (80.0241, -226.1679) centre (80.0241, -227.4359) cw
  line L215 (78.7561, -227.436) -> (78.7561, -237.58)
  arc A100 (140.3318, -253.889) -> (139.0638, -252.621) centre (140.3318, -252.621) cw
  line L216 (140.3318, -253.889) -> (150.4758, -253.889)
  arc A101 (151.7438, -252.6209) -> (150.4758, -253.889) centre (150.4758, -252.621) cw
  line L217 (151.7438, -252.6209) -> (151.7438, -242.4769)
  arc A102 (150.4758, -241.2089) -> (151.7438, -242.4769) centre (150.4758, -242.477) cw
  line L218 (150.4758, -241.2089) -> (140.3318, -241.2089)
  arc A103 (139.0638, -242.4769) -> (140.3318, -241.2089) centre (140.3318, -242.477) cw
  line L219 (139.0638, -242.4769) -> (139.0638, -252.621)
  arc A104 (125.3436, -253.9301) -> (124.0756, -252.662) centre (125.3436, -252.662) cw
  line L220 (125.3436, -253.9301) -> (135.4877, -253.9301)
  arc A105 (136.7557, -252.662) -> (135.4877, -253.9301) centre (135.4877, -252.662) cw
  line L221 (136.7557, -252.662) -> (136.7557, -242.518)
  arc A106 (135.4877, -241.25) -> (136.7557, -242.518) centre (135.4877, -242.518) cw
  line L222 (135.4877, -241.25) -> (125.3436, -241.25)
  arc A107 (124.0756, -242.518) -> (125.3436, -241.25) centre (125.3436, -242.518) cw
  line L223 (124.0756, -242.518) -> (124.0756, -252.662)
  arc A108 (110.2136, -253.9301) -> (108.9456, -252.662) centre (110.2136, -252.662) cw
  line L224 (110.2136, -253.9301) -> (120.3577, -253.9301)
  arc A109 (121.6257, -252.662) -> (120.3577, -253.9301) centre (120.3577, -252.662) cw
  line L225 (121.6257, -252.662) -> (121.6257, -242.518)
  arc A110 (120.3577, -241.25) -> (121.6257, -242.518) centre (120.3577, -242.518) cw
  line L226 (120.3577, -241.25) -> (110.2136, -241.25)
  arc A111 (108.9456, -242.518) -> (110.2136, -241.25) centre (110.2136, -242.518) cw
  line L227 (108.9456, -242.518) -> (108.9456, -252.662)
  arc A112 (95.0489, -253.9301) -> (93.7809, -252.662) centre (95.0489, -252.662) cw
  line L228 (95.0489, -253.9301) -> (105.193, -253.9301)
  arc A113 (106.461, -252.662) -> (105.193, -253.9301) centre (105.193, -252.662) cw
  line L229 (106.461, -252.662) -> (106.461, -242.518)
  arc A114 (105.193, -241.25) -> (106.461, -242.518) centre (105.193, -242.518) cw
  line L230 (105.193, -241.25) -> (95.0489, -241.25)
  arc A115 (93.7809, -242.518) -> (95.0489, -241.25) centre (95.0489, -242.518) cw
  line L231 (93.7809, -242.518) -> (93.7809, -252.662)
  arc A116 (80.0241, -253.9301) -> (78.756, -252.662) centre (80.0241, -252.662) cw
  line L232 (80.0241, -253.9301) -> (90.1681, -253.9301)
  arc A117 (91.4361, -252.662) -> (90.1681, -253.9301) centre (90.1681, -252.662) cw
  line L233 (91.4361, -252.662) -> (91.4361, -242.518)
  arc A118 (90.1681, -241.25) -> (91.4361, -242.518) centre (90.1681, -242.518) cw
  line L234 (90.1681, -241.25) -> (80.0241, -241.25)
  arc A119 (78.756, -242.518) -> (80.0241, -241.25) centre (80.0241, -242.518) cw
  line L235 (78.756, -242.518) -> (78.756, -252.662)
  arc A120 (160.8405, -250.3707) -> (165.8205, -250.3707) centre (163.3305, -250.3681) cw
  arc A121 (165.8205, -250.3707) -> (160.8405, -250.3707) centre (163.3305, -250.3734) cw
  ellipse E116 centre (26.873, -250.3909) end of major axis (29.3663, -250.3909) minor radius 2.492 (29.3663, -250.3909) -> (24.3798, -250.3909) cw
  ellipse E117 centre (26.873, -250.3909) end of major axis (29.3663, -250.3909) minor radius 2.492 (24.3798, -250.3909) -> (29.3663, -250.3909) cw
  ellipse E118 centre (163.3052, -155.0041) end of major axis (165.7973, -155.0041) minor radius 2.4899 (165.7973, -155.0041) -> (160.8131, -155.0041) cw
  ellipse E119 centre (163.3052, -155.0041) end of major axis (165.7973, -155.0041) minor radius 2.4899 (160.8131, -155.0041) -> (165.7973, -155.0041) cw
  arc A122 (24.3761, -154.9952) -> (29.3602, -154.9952) centre (26.8681, -154.9941) cw
  arc A123 (29.3602, -154.9952) -> (24.3761, -154.9952) centre (26.8681, -154.9963) cw
  ellipse E120 centre (163.2903, -50.1084) end of major axis (165.7824, -50.1084) minor radius 2.4899 (160.7982, -50.1106) -> (165.7824, -50.1106) cw
  ellipse E121 centre (163.2903, -50.1128) end of major axis (165.7824, -50.1128) minor radius 2.4899 (165.7824, -50.1106) -> (160.7982, -50.1106) cw
  ellipse E122 centre (26.863, -50.1096) end of major axis (29.3551, -50.1096) minor radius 2.4913 (24.371, -50.112) -> (29.3551, -50.112) cw
  ellipse E123 centre (26.863, -50.1145) end of major axis (29.3551, -50.1145) minor radius 2.4913 (29.3551, -50.112) -> (24.371, -50.112) cw
  ellipse E124 centre (153.6745, -109.7292) end of major axis (154.9767, -109.7292) minor radius 1.2936 (153.6745, -111.0228) -> (152.3723, -109.7291) cw
  line L236 (153.6745, -111.0228) -> (164.7434, -111.0228)
  ellipse E125 centre (164.7434, -109.7292) end of major axis (166.0456, -109.7292) minor radius 1.2936 (166.0456, -109.7291) -> (164.7434, -111.0228) cw
  line L237 (166.0456, -109.7291) -> (166.0456, -103.6491)
  ellipse E126 centre (164.7434, -103.6491) end of major axis (166.0456, -103.6491) minor radius 1.2936 (164.7434, -102.3554) -> (166.0456, -103.6491) cw
  line L238 (164.7434, -102.3554) -> (153.6745, -102.3554)
  ellipse E127 centre (153.6745, -103.6491) end of major axis (154.9767, -103.6491) minor radius 1.2936 (152.3723, -103.6491) -> (153.6745, -102.3554) cw
  line L239 (152.3723, -103.6491) -> (152.3723, -109.7291)
  line L240 (146.2625, -54.5555) -> (146.2625, -125.1966)
  spline S0 degree 3 poles (146.2625, -125.1966) (146.2625, -126.9557) (144.8465, -128.3718) (143.0874, -128.3718) knots 0 0 0 0 1 1 1 1
  line L241 (143.0874, -128.3718) -> (46.9155, -128.3718)
  spline S1 degree 3 poles (46.9155, -128.3718) (45.1564, -128.3718) (43.7403, -126.9557) (43.7403, -125.1966) knots 0 0 0 0 1 1 1 1
  line L242 (43.7403, -125.1966) -> (43.7403, -54.5555)
  spline S2 degree 3 poles (43.7403, -54.5555) (43.7403, -52.7963) (45.1564, -51.3798) (46.9155, -51.3798) knots 0 0 0 0 1 1 1 1
  line L243 (46.9155, -51.3798) -> (143.0874, -51.3798)
  spline S3 degree 3 poles (143.0874, -51.3798) (144.8465, -51.3798) (146.2625, -52.7963) (146.2625, -54.5555) knots 0 0 0 0 1 1 1 1
  line L244 (29.2103, -182.56) -> (33.0805, -182.56)
  spline S4 degree 3 poles (33.0805, -182.56) (34.1668, -182.56) (34.9816, -183.176) (34.9816, -183.8867) knots 0 0 0 0 1 1 1 1
  line L245 (34.9816, -183.8867) -> (34.9816, -234.9609)
  spline S5 degree 3 poles (34.9816, -234.9609) (34.9816, -235.7189) (34.0989, -236.2875) (33.0805, -236.2875) knots 0 0 0 0 1 1 1 1
  line L246 (33.0805, -236.2875) -> (29.2103, -236.2875)
  spline S6 degree 3 poles (29.2103, -236.2875) (28.1239, -236.2875) (27.3092, -235.6716) (27.3092, -234.9609) knots 0 0 0 0 1 1 1 1
  line L247 (27.3092, -234.9609) -> (27.3092, -183.934)
  spline S7 degree 3 poles (27.3092, -183.934) (27.3092, -183.176) (28.1239, -182.56) (29.2103, -182.56) knots 0 0 0 0 1 1 1 1
  line L248 (155.8034, -182.5597) -> (159.6736, -182.5597)
  spline S8 degree 3 poles (159.6736, -182.5597) (160.7599, -182.5597) (161.5747, -183.1757) (161.5747, -183.8863) knots 0 0 0 0 1 1 1 1
  line L249 (161.5747, -183.8863) -> (161.5747, -234.9606)
  spline S9 degree 3 poles (161.5747, -234.9606) (161.5747, -235.7186) (160.692, -236.2872) (159.6736, -236.2872) knots 0 0 0 0 1 1 1 1
  line L250 (159.6736, -236.2872) -> (155.8034, -236.2872)
  spline S10 degree 3 poles (155.8034, -236.2872) (154.717, -236.2872) (153.9023, -235.6712) (153.9023, -234.9606) knots 0 0 0 0 1 1 1 1
  line L251 (153.9023, -234.9606) -> (153.9023, -183.9337)
  spline S11 degree 3 poles (153.9023, -183.9337) (153.9023, -183.1756) (154.717, -182.5597) (155.8034, -182.5597) knots 0 0 0 0 1 1 1 1
  arc A124 (64.9191, -252.995) -> (63.8462, -251.9221) centre (64.9191, -251.9221) cw
  line L252 (64.9191, -252.995) -> (73.5025, -252.995)
  arc A125 (74.5755, -251.9221) -> (73.5025, -252.995) centre (73.5025, -251.9221) cw
  line L253 (74.5755, -251.9221) -> (74.5755, -243.3387)
  arc A126 (73.5025, -242.2658) -> (74.5755, -243.3387) centre (73.5025, -243.3387) cw
  line L254 (73.5025, -242.2658) -> (64.9191, -242.2658)
  arc A127 (63.8462, -243.3387) -> (64.9191, -242.2658) centre (64.9191, -243.3387) cw
  line L255 (63.8462, -243.3387) -> (63.8462, -251.9221)
  arc A128 (51.6032, -252.995) -> (50.5303, -251.9221) centre (51.6032, -251.9221) cw
  line L256 (51.6032, -252.995) -> (60.1866, -252.995)
  arc A129 (61.2596, -251.9221) -> (60.1866, -252.995) centre (60.1866, -251.9221) cw
  line L257 (61.2596, -251.9221) -> (61.2596, -243.3387)
  arc A130 (60.1866, -242.2658) -> (61.2596, -243.3387) centre (60.1866, -243.3387) cw
  line L258 (60.1866, -242.2658) -> (51.6032, -242.2658)
  arc A131 (50.5303, -243.3387) -> (51.6032, -242.2658) centre (51.6032, -243.3387) cw
  line L259 (50.5303, -243.3387) -> (50.5303, -251.9221)
  arc A132 (38.2293, -252.995) -> (37.1563, -251.9221) centre (38.2293, -251.9221) cw
  line L260 (38.2293, -252.995) -> (46.8127, -252.995)
  arc A133 (47.8856, -251.9221) -> (46.8127, -252.995) centre (46.8127, -251.9221) cw
  line L261 (47.8856, -251.9221) -> (47.8856, -243.3387)
  arc A134 (46.8127, -242.2658) -> (47.8856, -243.3387) centre (46.8127, -243.3387) cw
  line L262 (46.8127, -242.2658) -> (38.2293, -242.2658)
  arc A135 (37.1563, -243.3387) -> (38.2293, -242.2658) centre (38.2293, -243.3387) cw
  line L263 (37.1563, -243.3387) -> (37.1563, -251.9221)
  arc A136 (64.9191, -240.4595) -> (63.8462, -239.3866) centre (64.9191, -239.3866) cw
  line L264 (64.9191, -240.4595) -> (73.5025, -240.4595)
  arc A137 (74.5755, -239.3866) -> (73.5025, -240.4595) centre (73.5025, -239.3866) cw
  line L265 (74.5755, -239.3866) -> (74.5755, -230.8032)
  arc A138 (73.5025, -229.7303) -> (74.5755, -230.8032) centre (73.5025, -230.8032) cw
  line L266 (73.5025, -229.7303) -> (64.9191, -229.7303)
  arc A139 (63.8462, -230.8032) -> (64.9191, -229.7303) centre (64.9191, -230.8032) cw
  line L267 (63.8462, -230.8032) -> (63.8462, -239.3866)
  arc A140 (51.6032, -240.4595) -> (50.5303, -239.3866) centre (51.6032, -239.3866) cw
  line L268 (51.6032, -240.4595) -> (60.1866, -240.4595)
  arc A141 (61.2596, -239.3866) -> (60.1866, -240.4595) centre (60.1866, -239.3866) cw
  line L269 (61.2596, -239.3866) -> (61.2596, -230.8032)
  arc A142 (60.1866, -229.7303) -> (61.2596, -230.8032) centre (60.1866, -230.8032) cw
  line L270 (60.1866, -229.7303) -> (51.6032, -229.7303)
  arc A143 (50.5303, -230.8032) -> (51.6032, -229.7303) centre (51.6032, -230.8032) cw
  line L271 (50.5303, -230.8032) -> (50.5303, -239.3866)
  arc A144 (38.2293, -240.4595) -> (37.1563, -239.3866) centre (38.2293, -239.3866) cw
  line L272 (38.2293, -240.4595) -> (46.8127, -240.4595)
  arc A145 (47.8856, -239.3866) -> (46.8127, -240.4595) centre (46.8127, -239.3866) cw
  line L273 (47.8856, -239.3866) -> (47.8856, -230.8032)
  arc A146 (46.8127, -229.7303) -> (47.8856, -230.8032) centre (46.8127, -230.8032) cw
  line L274 (46.8127, -229.7303) -> (38.2293, -229.7303)
  arc A147 (37.1563, -230.8032) -> (38.2293, -229.7303) centre (38.2293, -230.8032) cw
  line L275 (37.1563, -230.8032) -> (37.1563, -239.3866)
  arc A148 (64.9191, -227.7443) -> (63.8462, -226.6714) centre (64.9191, -226.6714) cw
  line L276 (64.9191, -227.7443) -> (73.5025, -227.7443)
  arc A149 (74.5755, -226.6714) -> (73.5025, -227.7443) centre (73.5025, -226.6714) cw
  line L277 (74.5755, -226.6714) -> (74.5755, -218.088)
  arc A150 (73.5025, -217.0151) -> (74.5755, -218.088) centre (73.5025, -218.088) cw
  line L278 (73.5025, -217.0151) -> (64.9191, -217.0151)